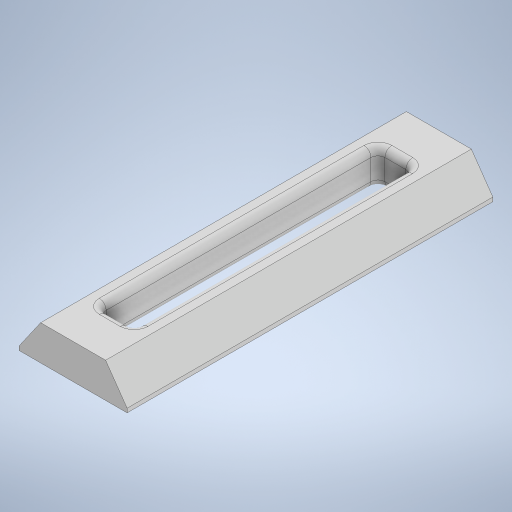
# Autodesk Inventor part: esercizio3 02-27-2023
Saved by Autodesk Inventor 2023 (Build 270158000, 158)
## iProperties
Created: 2023-02-27
Part Number: esercizio3 02-27-2023
Material: Generico
Document SubType Name: Modeling
Designer: Admin
Density: 1 g/cm^3
Appearance: Default
Author: Admin
Autodesk Inventor part; units mm, degrees
ref_plane "YZ Plane" through (0, 0, 0) normal (1, 0, 0) x (0, 1, 0)
ref_plane "XZ Plane" through (0, 0, 0) normal (0, 1, 0) x (-1, 0, 0)
ref_plane "XY Plane" through (0, 0, 0) normal (0, 0, 1) x (1, 0, 0)
sketch "Schizzo1" plane through (0, 0, 0) normal (0, 0, 1) x (1, 0, 0)
  line L0 (-8.5308, -2.9405) -> (22.4692, -2.9405)
  line L1 (22.4692, -2.9405) -> (22.4692, -1.7792)
  line L2 (22.4692, -1.7792) -> (16.2975, 7.0595)
  line L3 (-2.3591, 7.0595) -> (-8.5308, -1.7792)
  line L4 (-8.5308, -1.7792) -> (-8.5308, -2.9405)
  line L5 (6.9692, 7.0595) -> (6.9692, -2.9405)
  line L6 (6.9692, 7.0595) -> (27.9692, 7.0595) construction
  line L7 (27.9692, 7.0595) -> (23.9692, 7.0595) construction
  line L8 (23.9692, 7.0595) -> (23.9692, 3.0595) construction
  circle A0 centre (23.9692, 3.0595) radius 4 construction
  line L9 (6.9692, 7.0595) -> (-14.0308, 7.0595) construction
  line L10 (-14.0308, 7.0595) -> (-10.0308, 7.0595) construction
  line L11 (-10.0308, 7.0595) -> (-10.0308, 3.0595) construction
  circle A1 centre (-10.0308, 3.0595) radius 4 construction
  line L12 (-2.3591, 7.0595) -> (16.2975, 7.0595)
  dimension "d1" = 31
  dimension "d6" = 10
  dimension "d7" = 21
  dimension "d8" = 4
  dimension "d9" = 4
  dimension "d10" = 10
  dimension "d11" = 21
  dimension "d12" = 4
  dimension "d13" = 4
  constraints: 26 end point, 3 horizontal, 3 perpendicular, 3 point on line, 2 coincident, 2 vertical alignment, 1 midpoint, 1 vertical, 7 other
  measures "d1" distance of L0.start L0.end
  measures "d6" distance from line of L0 L2.end
  measures "d7" distance of L5.start L6.end
  measures "d8" distance of L6.end L7.end
  measures "d9" distance of L7.end L8.end
  measures "d10" distance between parallel lines of L0 L6
  measures "d11" distance of L5.start L9.end
  measures "d12" distance of L9.end L10.end
  measures "d13" distance of L10.end L11.end
extrude "Estrusione1" add sketch "Schizzo1" along normal mid plane 105
sketch "Schizzo3" plane through (-2.3591, 7.0595, 52.5) normal (0, 1, 0) x (1, 0, 0)
  line L0 (18.6566, 0) -> (0, 0) projected
  line L1 (0, 52.5) -> (18.6566, 52.5) construction
  line L2 (18.6566, 0) -> (18.6566, 105) projected
  line L3 (0, 0) -> (9.3283, 0)
  line L4 (9.3283, 0) -> (9.3283, 105) construction
  line L5 (24.8283, 105) -> (-6.1717, 105) projected
  line L6 (9.3283, 92.5) -> (4.3283, 92.5)
  line L7 (4.3283, 92.5) -> (4.3283, 12.5)
  line L8 (4.3283, 12.5) -> (14.3283, 12.5)
  line L9 (14.3283, 12.5) -> (14.3283, 92.5)
  line L10 (14.3283, 92.5) -> (9.3283, 92.5)
  point P0 (2.3591, 52.5)
  dimension "d18" = 5
  dimension "d19" = 80
  dimension "d20" = 10
  constraints: 16 end point, 4 perpendicular, 3 midpoint, 2 point on line
  measures "d18" distance of L6.start L6.end
  measures "d19" distance of L6.end L7.end
  measures "d20" distance of L7.end L8.end
extrude "Estrusione2" cut sketch "Schizzo3" against normal blind 10
fillet "Raccordo1" radius 2 8 edges at (11.9692, 2.0595, 40) (1.9692, 2.0595, 40) (1.9692, 2.0595, -40) (11.9692, 2.0595, -40) (11.9692, 7.0595, 0) (1.9692, 7.0595, 0) (6.9692, 7.0595, -40) (6.9692, 7.0595, 40)
fillet "Raccordo2" radius 2 8 edges at (11.3834, -2.9405, -39.4142) (6.9692, -2.9405, -40) (2.555, -2.9405, -39.4142) (1.9692, -2.9405, 0) (2.555, -2.9405, 39.4142) (6.9692, -2.9405, 40) (11.3834, -2.9405, 39.4142) (11.9692, -2.9405, 0)
